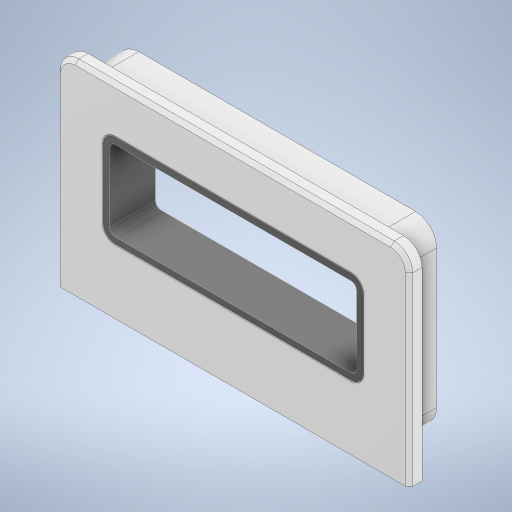
# Autodesk Inventor part: Door Handle
Saved by Autodesk Inventor 2024 (Build 280153000, 153)
## iProperties
Created: 2024-12-01
Part Number: Door Handle
Material: ABS Plastic
Document SubType Name: Modeling
Designer: Ishaan
Density: 1.06 g/cm^3
Appearance: Smooth - Black
Author: Ishaan
Autodesk Inventor part; units mm, degrees
sketch "Sketch1" plane through (0, 0, 0) normal (0, 0, 1) x (1, 0, 0)
  line L0 (75, -37.5) -> (-75, -37.5) construction
  line L1 (-75, -37.5) -> (-75, 37.5) construction
  line L2 (-75, 37.5) -> (75, 37.5) construction
  line L3 (75, 37.5) -> (75, -37.5) construction
  line L4 (75, -37.5) -> (-75, 37.5) construction
  line L5 (-75, -37.5) -> (75, 37.5) construction
  line L6 (75, 45.5) -> (-75, 45.5)
  line L7 (-83, 37.5) -> (-83, -37.5)
  line L8 (-75, -45.5) -> (75, -45.5)
  line L9 (83, -37.5) -> (83, 37.5)
  arc A0 (-75, 45.5) -> (-83, 37.5) centre (-75, 37.5) ccw
  arc A1 (83, 37.5) -> (75, 45.5) centre (75, 37.5) ccw
  arc A2 (75, -45.5) -> (83, -37.5) centre (75, -37.5) ccw
  arc A3 (-83, -37.5) -> (-75, -45.5) centre (-75, -37.5) ccw
  point P0 (0, 0)
  dimension "d0" = 150
  dimension "d1" = 75
  dimension "d3" = 8
  constraints: 20 end point, 8 point on circle, 8 tangent, 4 centre point, 4 parallel, 3 equal radius, 2 midpoint, 2 perpendicular, 1 coincident, 1 horizontal, 3 other
  measures "d0" distance of L1.end L2.end
  measures "d1" distance of L2.end L0.start
  measures "d3" distance between parallel lines of L6 L2
extrude "Extrusion1" add sketch "Sketch1" along normal blind 25
sketch "Sketch2" plane through (0, 0, 25) normal (0, 0, 1) x (1, 0, 0)
  line L0 (67, -20.5) -> (-67, -20.5)
  line L1 (-67, -20.5) -> (-67, 29.5)
  line L2 (-67, 29.5) -> (67, 29.5)
  line L3 (67, 29.5) -> (67, -20.5)
  line L4 (67, -20.5) -> (-67, 29.5) construction
  line L5 (-67, -20.5) -> (67, 29.5) construction
  line L6 (75, 45.5) -> (-75, 45.5) projected
  line L7 (-83, 37.5) -> (-83, -37.5) projected
  point P0 (0, 0)
  point P1 (0, 4.5)
  point P2 (0, 29.5)
  dimension "d6" = 16
  dimension "d7" = 16
  dimension "d8" = 50
  constraints: 12 end point, 3 midpoint, 2 parallel, 1 horizontal, 1 perpendicular, 1 vertical alignment
  measures "d6" distance between parallel lines of L6 L2
  measures "d7" distance between parallel lines of L1 L7
  measures "d8" distance of L2.end L0.start
extrude "Extrusion2" cut sketch "Sketch2" against normal through all
sketch "Sketch3" plane through (0, 0, 0) normal (1, 0, 0) x (0, 1, 0)
  line L0 (45.5, 25) -> (45.5, 0) projected
  line L1 (45.5, 0) -> (29.5, 0) projected
  line L2 (29.5, 0) -> (29.5, 25) projected
  line L3 (29.5, 25) -> (45.5, 25) projected
  line L4 (-45.5, 0) -> (-45.5, 25) projected
  line L5 (-45.5, 25) -> (-20.5, 25) projected
  line L6 (-20.5, 25) -> (-20.5, 0) projected
  line L7 (-20.5, 0) -> (-45.5, 0) projected
  line L8 (29.5, 25) -> (22.8013, 25)
  line L9 (37.5, 25) -> (-37.5, 25) projected
  line L10 (29.5, 0) -> (22.8013, 25)
  point P0 (0, 0)
  dimension "d12" = 15
  constraints: 4 end point, 1 point on line
  measures "d12" angle of L2 L10
extrude "Extrusion3" add sketch "Sketch3" along normal up to surface (134 mm away) from surface at -67 contours L10 L8 L2
fillet "Fillet1" radius 3 4 edges at (-67, 26.1506, 12.5) (-67, -20.5, 12.5) (67, -20.5, 12.5) (67, 26.1506, 12.5)
sketch "Sketch4" plane through (0, 0, 25) normal (0, 0, 1) x (1, 0, 0)
  line L0 (-67, -17.5) -> (-67, 19.6954) projected
  ellipse E0 centre (-64, 19.6954) end of major axis (-64, 22.8013) minor radius 3 (-64, 22.8013) -> (-67, 19.6954) ccw projected
  line L1 (-64, 22.8013) -> (64, 22.8013) projected
  ellipse E1 centre (64, 19.6954) end of major axis (64, 22.8013) minor radius 3 (67, 19.6954) -> (64, 22.8013) ccw projected
  line L2 (67, 19.6954) -> (67, -17.5) projected
  arc A0 (64, -20.5) -> (67, -17.5) centre (64, -17.5) ccw projected
  line L3 (64, -20.5) -> (-64, -20.5) projected
  arc A1 (-67, -17.5) -> (-64, -20.5) centre (-64, -17.5) ccw projected
  arc A2 (-75, 45.5) -> (-83, 37.5) centre (-75, 37.5) ccw projected
  line L4 (-83, 37.5) -> (-83, -37.5) projected
  arc A3 (-83, -37.5) -> (-75, -45.5) centre (-75, -37.5) ccw projected
  line L5 (-75, -45.5) -> (75, -45.5) projected
  arc A4 (75, -45.5) -> (83, -37.5) centre (75, -37.5) ccw projected
  line L6 (83, -37.5) -> (83, 37.5) projected
  arc A5 (83, 37.5) -> (75, 45.5) centre (75, 37.5) ccw projected
  line L7 (75, 45.5) -> (-75, 45.5) projected
  line L8 (64, 26.3013) -> (-64, 26.3013)
  line L9 (-70.5, 19.6954) -> (-70.5, -17.5)
  arc A6 (-70.5, -17.5) -> (-64, -24) centre (-64, -17.5) ccw
  line L10 (-64, -24) -> (64, -24)
  arc A7 (64, -24) -> (70.5, -17.5) centre (64, -17.5) ccw
  line L11 (70.5, -17.5) -> (70.5, 19.6954)
  spline S0 degree 5 poles (-64, 26.3013) (-65.0362, 26.3013) (-66.0724, 26.0915) (-67.0518, 25.6717) (-68.7744, 24.4734) (-69.9162, 22.7138) (-70.3054, 21.7405) (-70.5, 20.7179) (-70.5, 19.6954) knots 0 0 0 0 0 0 0.503323 0.503323 0.503323 1 1 1 1 1 1
  spline S1 degree 5 poles (70.5, 19.6954) (70.5, 20.7179) (70.3054, 21.7405) (69.9162, 22.7138) (68.7744, 24.4734) (67.0518, 25.6717) (66.0724, 26.0915) (65.0362, 26.3013) (64, 26.3013) knots 0 0 0 0 0 0 0.496677 0.496677 0.496677 1 1 1 1 1 1
  point P0 (0, 0)
  dimension "d16" = 3.5
  constraints: 8 end point, 4 point on circle, 3 parallel, 2 centre point, 12 other
  measures "d16" distance between parallel lines of L1 L8
extrude "Extrusion4" cut sketch "Sketch4" against normal blind 3.4 contours L7 A5 L6 A4 L5 A3 L4 A2
ref_plane "Work Plane1" through (0, 0, 8) normal (0, 0, -1) x (-1, 0, 0)
sketch "Sketch5" plane through (0, 0, 8) normal (0, 0, -1) x (-1, 0, 0)
  line L0 (-75, 37.5) -> (-75, -37.5) construction
  line L1 (75, 37.5) -> (-75, 37.5) construction
  line L2 (75, -37.5) -> (75, 37.5) construction
  line L3 (-75, -37.5) -> (75, -37.5) construction
  point P0 (0, 0)
  point P1 (0, 37.5)
  point P2 (0, -37.5)
  constraints: 4 coincident, 2 midpoint
hole "Hole1" at (-75, 37.5, 8) at (0, 37.5, 8) at (75, 37.5, 8) at (75, -37.5, 8) at (0, -37.5, 8) at (-75, -37.5, 8) direction (0, 0, -1) diameter 5.4 end through all both
hole "Hole2" at (-75, -37.5, 8) at (0, -37.5, 8) at (75, -37.5, 8) direction (0, 0, 1) diameter 9.5 end through all
sketch "Sketch6" plane through (0, 0, 25) normal (0, 0, 1) x (1, 0, 0)
  line L0 (70.5, -17.5) -> (70.5, 19.6954) projected
  spline S0 degree 5 poles (70.5, 19.6954) (70.5, 20.7179) (70.3054, 21.7405) (69.9162, 22.7138) (68.7744, 24.4734) (67.0518, 25.6717) (66.0724, 26.0915) (65.0362, 26.3013) (64, 26.3013) knots 0 0 0 0 0 0 0.496677 0.496677 0.496677 1 1 1 1 1 1
  line L1 (64, 26.3013) -> (-64, 26.3013) projected
  spline S1 degree 5 poles (-64, 26.3013) (-65.0362, 26.3013) (-66.0724, 26.0915) (-67.0518, 25.6717) (-68.7744, 24.4734) (-69.9162, 22.7138) (-70.3054, 21.7405) (-70.5, 20.7179) (-70.5, 19.6954) knots 0 0 0 0 0 0 0.503323 0.503323 0.503323 1 1 1 1 1 1
  line L2 (-70.5, 19.6954) -> (-70.5, -17.5) projected
  arc A0 (-70.5, -17.5) -> (-64, -24) centre (-64, -17.5) ccw projected
  line L3 (-64, -24) -> (64, -24) projected
  arc A1 (64, -24) -> (70.5, -17.5) centre (64, -17.5) ccw projected
  line L4 (-67, -17.5) -> (-67, 19.6954) projected
  ellipse E0 centre (-64, 19.6954) end of major axis (-64, 22.8013) minor radius 3 (-64, 22.8013) -> (-67, 19.6954) ccw projected
  line L5 (-64, 22.8013) -> (64, 22.8013) projected
  ellipse E1 centre (64, 19.6954) end of major axis (64, 22.8013) minor radius 3 (67, 19.6954) -> (64, 22.8013) ccw projected
  line L6 (67, 19.6954) -> (67, -17.5) projected
  arc A2 (64, -20.5) -> (67, -17.5) centre (64, -17.5) ccw projected
  line L7 (64, -20.5) -> (-64, -20.5) projected
  arc A3 (-67, -17.5) -> (-64, -20.5) centre (-64, -17.5) ccw projected
  line L8 (-64, 26.7013) -> (64, 26.7013)
  line L9 (70.9, 19.6954) -> (70.9, -17.5)
  arc A4 (64, -24.4) -> (70.9, -17.5) centre (64, -17.5) ccw
  line L10 (64, -24.4) -> (-64, -24.4)
  arc A5 (-70.9, -17.5) -> (-64, -24.4) centre (-64, -17.5) ccw
  line L11 (-70.9, -17.5) -> (-70.9, 19.6954)
  line L12 (95.5, -58.85) -> (-95.5, -58.85)
  line L13 (-95.5, -58.85) -> (-95.5, 51.3013)
  line L14 (-95.5, 51.3013) -> (95.5, 51.3013)
  line L15 (95.5, 51.3013) -> (95.5, -58.85)
  line L16 (95.5, -58.85) -> (-95.5, 51.3013) construction
  line L17 (-95.5, -58.85) -> (95.5, 51.3013) construction
  line L18 (75, -45.5) -> (-75, -45.5) projected
  spline S2 degree 5 poles (-70.9, 19.6954) (-70.8989, 21.8801) (-70.0664, 24.0626) (-68.3751, 25.8251) (-66.183, 26.7011) (-64, 26.7013) knots 0 0 0 0 0 0 1 1 1 1 1 1
  spline S3 degree 5 poles (64, 26.7013) (66.183, 26.7011) (68.3751, 25.8251) (70.0664, 24.0626) (70.8989, 21.8801) (70.9, 19.6954) knots 0 0 0 0 0 0 1 1 1 1 1 1
  point P0 (0, 0)
  point P1 (0, -3.7744)
  point P2 (0, 51.3013)
  dimension "d34" = 0.4
  dimension "d35" = 25
  dimension "d36" = 25
  dimension "d37" = 13.35
  constraints: 20 end point, 5 parallel, 4 point on circle, 3 midpoint, 2 centre point, 1 horizontal, 1 perpendicular, 1 vertical alignment, 14 other
  measures "d35" distance between parallel lines of L13 L2
  measures "d36" distance between parallel lines of L14 L1
  measures "d37" distance between parallel lines of L18 L12
extrude "Extrusion5" add sketch "Sketch6" against normal blind 3 separate body contours L12 L13 L14 L15
fillet "Fillet2" radius 10 2 edges at (-95.5, 51.3013, 23.5) (95.5, 51.3013, 23.5)
sketch "Sketch7" plane through (0, 0, 22) normal (0, 0, -1) x (-1, 0, 0)
  circle A0 centre (75, -37.5) radius 2.7 projected
  circle A1 centre (0, -37.5) radius 2.7 projected
  circle A2 centre (-75, -37.5) radius 2.7 projected
  circle A3 centre (-75, 37.5) radius 2.7 projected
  circle A4 centre (0, 37.5) radius 2.7 projected
  circle A5 centre (75, 37.5) radius 2.7 projected
  line L0 (67, 26.3942) -> (67, -17.5) projected
  arc A6 (64, -20.5) -> (67, -17.5) centre (64, -17.5) ccw projected
  line L1 (64, -20.5) -> (-64, -20.5) projected
  arc A7 (-67, -17.5) -> (-64, -20.5) centre (-64, -17.5) ccw projected
  line L2 (-67, -17.5) -> (-67, 26.3942) projected
  ellipse E0 centre (-64, 26.3942) end of major axis (-64, 29.5) minor radius 3 (-64, 29.5) -> (-67, 26.3942) ccw projected
  line L3 (-64, 29.5) -> (64, 29.5) projected
  ellipse E1 centre (64, 26.3942) end of major axis (64, 29.5) minor radius 3 (67, 26.3942) -> (64, 29.5) ccw projected
  arc A8 (83, 37.5) -> (75, 45.5) centre (75, 37.5) ccw projected
  line L4 (-75, 45.5) -> (75, 45.5) projected
  arc A9 (-75, 45.5) -> (-83, 37.5) centre (-75, 37.5) ccw projected
  line L5 (-83, -37.5) -> (-83, 37.5) projected
  arc A10 (-83, -37.5) -> (-75, -45.5) centre (-75, -37.5) ccw projected
  line L6 (75, -45.5) -> (-75, -45.5) projected
  arc A11 (75, -45.5) -> (83, -37.5) centre (75, -37.5) ccw projected
  line L7 (83, 37.5) -> (83, -37.5) projected
  arc A12 (-85.5, 51.3013) -> (-95.5, 41.3013) centre (-85.5, 41.3013) ccw projected
  line L8 (-95.5, 41.3013) -> (-95.5, -58.85) projected
  line L9 (-95.5, -58.85) -> (95.5, -58.85) projected
  line L10 (95.5, -58.85) -> (95.5, 41.3013) projected
  arc A13 (95.5, 41.3013) -> (85.5, 51.3013) centre (85.5, 41.3013) ccw projected
  line L11 (85.5, 51.3013) -> (-85.5, 51.3013) projected
  line L12 (70.9, 19.6954) -> (70.9, -17.5) projected
  arc A14 (64, -24.4) -> (70.9, -17.5) centre (64, -17.5) ccw projected
  line L13 (64, -24.4) -> (-64, -24.4) projected
  arc A15 (-70.9, -17.5) -> (-64, -24.4) centre (-64, -17.5) ccw projected
  line L14 (-70.9, -17.5) -> (-70.9, 19.6954) projected
  line L15 (-64, 26.7013) -> (64, 26.7013) projected
  arc A16 (83.4, 37.5) -> (75, 45.9) centre (75, 37.5) ccw
  line L16 (83.4, 37.5) -> (83.4, -37.5)
  arc A17 (75, -45.9) -> (83.4, -37.5) centre (75, -37.5) ccw
  line L17 (75, -45.9) -> (-75, -45.9)
  arc A18 (-83.4, -37.5) -> (-75, -45.9) centre (-75, -37.5) ccw
  line L18 (-83.4, -37.5) -> (-83.4, 37.5)
  arc A19 (-75, 45.9) -> (-83.4, 37.5) centre (-75, 37.5) ccw
  line L19 (-75, 45.9) -> (75, 45.9)
  point P0 (0, 0)
  dimension "d41" = 0.4
  constraints: 8 end point, 8 point on circle, 4 centre point, 11 other
  measures "d41" distance between parallel lines of L4 L19
extrude "Extrusion6" add sketch "Sketch7" along normal blind 4 contours L11 A13 L10 L9 L8 A12 bodies 2
ref_plane "Work Plane2" through (0, 0, 1) normal (0, 0, -1) x (-1, 0, 0)
sketch "Sketch9" plane through (0, 0, 18) normal (0, 0, -1) x (-1, 0, 0)
  line L0 (-95.5, 41.3013) -> (-95.5, -58.85) projected
  line L1 (-95.5, -58.85) -> (95.5, -58.85) projected
  line L2 (95.5, -58.85) -> (95.5, 41.3013) projected
  arc A0 (95.5, 41.3013) -> (85.5, 51.3013) centre (85.5, 41.3013) ccw projected
  line L3 (85.5, 51.3013) -> (-85.5, 51.3013) projected
  arc A1 (-85.5, 51.3013) -> (-95.5, 41.3013) centre (-85.5, 41.3013) ccw projected
  line L4 (75, -45.9) -> (-75, -45.9) projected
  arc A2 (-83.4, -37.5) -> (-75, -45.9) centre (-75, -37.5) ccw projected
  line L5 (-83.4, -37.5) -> (-83.4, 37.5) projected
  arc A3 (-75, 45.9) -> (-83.4, 37.5) centre (-75, 37.5) ccw projected
  line L6 (-75, 45.9) -> (75, 45.9) projected
  arc A4 (83.4, 37.5) -> (75, 45.9) centre (75, 37.5) ccw projected
  line L7 (83.4, 37.5) -> (83.4, -37.5) projected
  arc A5 (75, -45.9) -> (83.4, -37.5) centre (75, -37.5) ccw projected
  line L8 (75, 48.9) -> (-75, 48.9)
  arc A6 (-75, 48.9) -> (-86.4, 37.5) centre (-75, 37.5) ccw
  line L9 (-86.4, 37.5) -> (-86.4, -37.5)
  arc A7 (-86.4, -37.5) -> (-75, -48.9) centre (-75, -37.5) ccw
  line L10 (-75, -48.9) -> (75, -48.9)
  arc A8 (75, -48.9) -> (86.4, -37.5) centre (75, -37.5) ccw
  line L11 (86.4, -37.5) -> (86.4, 37.5)
  arc A9 (86.4, 37.5) -> (75, 48.9) centre (75, 37.5) ccw
  point P0 (0, 0)
  dimension "d52" = 3
  constraints: 8 end point, 8 point on circle, 4 centre point, 7 other
  measures "d52" distance between parallel lines of L6 L8
extrude "Extrusion8" add sketch "Sketch9" along normal up to surface (17 mm away) contours A9 L11 A8 L10 A7 L9 A6 L8 bodies 2
fillet "Fillet3" radius 2 8 edges at (0, 48.9, 18) (-83.061, 45.561, 18) (-86.4, 0, 18) (-83.061, -45.561, 18) (0, -48.9, 18) (83.061, -45.561, 18) (86.4, 0, 18) (83.061, 45.561, 18)
chamfer "Chamfer3" distance 2 angle 45 5 edges at (95.5, -8.7744, 25) (92.5711, 48.3723, 25) (0, 51.3013, 25) (-92.5711, 48.3723, 25) (-95.5, -8.7744, 25)
ref_plane "Work Plane3" through (0, 0, 11) normal (0, 0, -1) x (-1, 0, 0)
sketch "Sketch11" plane through (0, 0, 11) normal (0, 0, -1) x (-1, 0, 0)
  circle A0 centre (-75, 37.5) radius 2.7 projected
  circle A1 centre (0, 37.5) radius 2.7 projected
  circle A2 centre (75, 37.5) radius 2.7 projected
  line L0 (72.6184, 41.625) -> (77.3816, 41.625)
  line L1 (77.3816, 41.625) -> (79.7631, 37.5)
  line L2 (79.7631, 37.5) -> (77.3816, 33.375)
  line L3 (77.3816, 33.375) -> (72.6184, 33.375)
  line L4 (72.6184, 33.375) -> (70.2369, 37.5)
  line L5 (70.2369, 37.5) -> (72.6184, 41.625)
  line L6 (-2.3816, 41.625) -> (2.3816, 41.625)
  line L7 (2.3816, 41.625) -> (4.7631, 37.5)
  line L8 (4.7631, 37.5) -> (2.3816, 33.375)
  line L9 (2.3816, 33.375) -> (-2.3816, 33.375)
  line L10 (-2.3816, 33.375) -> (-4.7631, 37.5)
  line L11 (-4.7631, 37.5) -> (-2.3816, 41.625)
  line L12 (-70.2369, 37.5) -> (-72.6184, 33.375)
  line L13 (-72.6184, 33.375) -> (-77.3816, 33.375)
  line L14 (-77.3816, 33.375) -> (-79.7631, 37.5)
  line L15 (-79.7631, 37.5) -> (-77.3816, 41.625)
  line L16 (-77.3816, 41.625) -> (-72.6184, 41.625)
  line L17 (-72.6184, 41.625) -> (-70.2369, 37.5)
  point P0 (0, 0)
  dimension "d60" = 8.25
  constraints: 36 end point, 3 coincident, 3 horizontal, 2 collinear, 39 other
  measures "d60" distance between parallel lines of L3 L0
extrude "Extrusion9" cut sketch "Sketch11" against normal through all contours A0 | A1 | A2 | L0 L1 L2 L3 L4 L5 | L6 L7 L8 L9 L10 L11 | L12 L13 L14 L15 L16 L17 bodies 1
equation "\"d7\" = d6"
equation "\"d36\" = d35"
body "Solid1"
